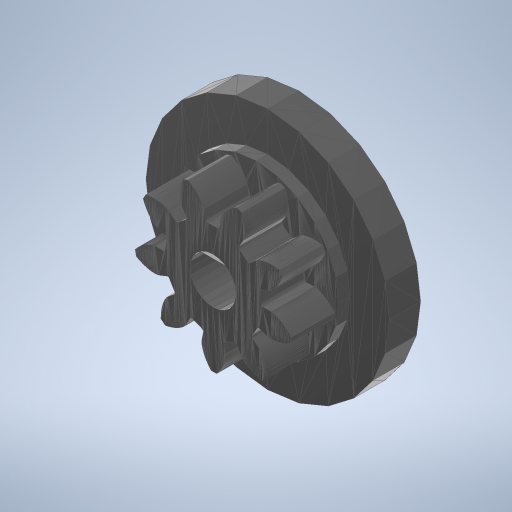
# Autodesk Inventor part: 6a_gear_100
Saved by Autodesk Inventor 2023.2 (Build 272271000, 271)
## iProperties
Created: 2023-03-13
Part Number: 6a_gear_100
Material: Generisch
Document SubType Name: Modeling
Designer: hangel
Density: 1 g/cm^3
Appearance: Vorgabe
Author: hangel
Autodesk Inventor part; units mm, degrees
ref_plane "YZ Plane" through (0, 0, 0) normal (1, 0, 0) x (0, 1, 0)
ref_plane "XZ Plane" through (0, 0, 0) normal (0, 1, 0) x (-1, 0, 0)
ref_plane "XY Plane" through (0, 0, 0) normal (0, 0, 1) x (1, 0, 0)
sketch "Skizze1" plane through (6.2367, -127.8831, -95.9414) normal (0, 0, 1) x (1, 0, 0)
  circle A0 centre (-6.5087, -2.3889) radius 2.52 projected
  line L0 (7.8366, -0.2889) -> (-23.4139, -0.2889)
  point P0 (-6.2367, 127.8831)
  point P1 (-7.9017, -0.2889)
  point P2 (-5.1157, -0.2889)
  dimension "d0" = 2.1
  constraints: 2 end point, 1 horizontal
  measures "d0" distance from line of L0 A0.centre
extrude "Extrusion1" add sketch "Skizze1" against normal blind 9.4 contours L0 A0 picked at (-6.2196, -0.2002)
